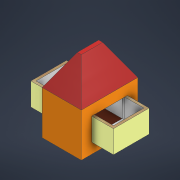
# Autodesk Inventor part: 110033226_ipt_55_內城堡屋頂
Saved by Autodesk Inventor 2022 (Build 260153000, 153)
## iProperties
Created: 2022-07-01
Part Number: 110033226_ipt_55_內城堡屋頂
Material: 一般
Document SubType Name: Modeling
Designer: User
Density: 1 g/cm^3
Appearance: 預設
Author: User
Autodesk Inventor part; units mm, degrees
ref_plane "YZ Plane" through (0, 0, 0) normal (1, 0, 0) x (0, 1, 0)
ref_plane "XZ Plane" through (0, 0, 0) normal (0, 1, 0) x (-1, 0, 0)
sketch "草圖1" plane through (0, 0, 0) normal (0, 1, 0) x (-1, 0, 0)
  line L0 (0, 0) -> (45, 0)
  line L1 (45, 0) -> (45, -65)
  line L2 (45, -65) -> (0, -65)
  line L3 (0, -65) -> (0, 0)
  dimension "d0" = 45
  dimension "d1" = 65
  constraints: 8 end point, 2 parallel, 1 horizontal, 1 perpendicular
  measures "d0" distance of L1.end L2.end
  measures "d1" distance of L0.end L1.end
extrude "擠出1" add sketch "草圖1" along normal blind 50
shell "薄殼1" thickness 3 removed faces 1 at (-15, 50, -21.666667)
sketch "草圖2" plane through (0, 0, 0) normal (1, 0, 0) x (0, 0, -1)
  line L0 (65, 50) -> (65, 0) projected
  line L1 (65, 0) -> (0, 0) projected
  line L2 (0, 0) -> (0, 50) projected
  line L3 (0, 50) -> (65, 50) projected
  line L4 (53, 38) -> (53, 12)
  line L5 (53, 12) -> (12, 12)
  line L6 (12, 12) -> (12, 38)
  line L7 (12, 38) -> (53, 38)
  dimension "d5" = 12
  constraints: 8 end point, 3 other
  measures "d5" distance between parallel lines of L3 L7
extrude "擠出2" add sketch "草圖2" along normal blind 25 separate body contours L4 L5 L6 L7
shell "薄殼2" thickness 3 removed faces 1 at (8.333333, 38, -39.333333) bodies 2
ref_plane "工作平面1" through (-22.5, 0, 0) normal (1, 0, 0) x (0, 0, -1)
sketch "草圖3" plane through (3, 15, -15) normal (1, 0, 0) x (0, 0, -1)
  line L0 (35, 0) -> (35, 23) projected
  line L1 (0, 23) -> (35, 23) projected
  line L2 (-3, 23) -> (0, 23) projected
  line L3 (-3, -3) -> (-3, 23) projected
  line L4 (38, -3) -> (-3, -3) projected
  line L5 (38, 23) -> (38, -3) projected
  line L6 (35, 23) -> (38, 23) projected
  line L7 (0, 0) -> (35, 0) projected
  line L8 (0, 23) -> (0, 0) projected
  point P0 (-15, -15)
extrude "擠出3" cut sketch "草圖3" against normal blind 25 contours L7 L8 L1 L0 bodies 2
sketch "草圖4" plane through (0, 0, 0) normal (1, 0, 0) x (0, 0, -1)
  line L0 (65, 50) -> (65, 0) projected
  line L1 (65, 0) -> (0, 0) projected
  line L2 (0, 0) -> (0, 50) projected
  line L3 (0, 50) -> (65, 50) projected
  line L4 (50, 38) -> (53, 38) projected
  line L5 (53, 38) -> (53, 12) projected
  line L6 (53, 12) -> (12, 12) projected
  line L7 (12, 12) -> (12, 38) projected
  line L8 (12, 38) -> (15, 38) projected
  line L9 (15, 38) -> (15, 15) projected
  line L10 (15, 15) -> (50, 15) projected
  line L11 (50, 15) -> (50, 38) projected
  line L12 (15, 38) -> (50, 38)
  line L13 (50, 38) -> (50, 15)
  line L14 (50, 15) -> (15, 15)
  line L15 (15, 15) -> (15, 38)
  constraints: 8 end point, 2 parallel, 1 horizontal, 1 perpendicular
extrude "擠出4" cut sketch "草圖4" against normal blind 10 contours L11 L10 L9 L12 bodies 1
mirror "鏡射1" about plane through (-22.5, 0, 0) normal (1, 0, 0) of "擠出4", "擠出2", "擠出3" bodies 1
shell "薄殼3" thickness 3 removed faces 1 at (-62.666667, 38, -26.666667) bodies 1
sketch "草圖5" plane through (-51, 15, -15) normal (-1, 0, 0) x (0, 0, 1)
  line L0 (0, 0) -> (0, 23) projected
  line L1 (-35, 23) -> (0, 23) projected
  line L2 (-38, 23) -> (-35, 23) projected
  line L3 (-38, -3) -> (-38, 23) projected
  line L4 (3, -3) -> (-38, -3) projected
  line L5 (3, 23) -> (3, -3) projected
  line L6 (0, 23) -> (3, 23) projected
  line L7 (-35, 0) -> (0, 0) projected
  line L8 (-35, 23) -> (-35, 0) projected
  point P0 (15, -15)
extrude "擠出5" cut sketch "草圖5" against normal blind 10 contours L7 L8 L1 L0 bodies 1
sketch "草圖6" plane through (0, 50, 0) normal (0, 1, 0) x (1, 0, 0)
  line L0 (-3, 3) -> (-3, 62) projected
  line L1 (-3, 62) -> (-42, 62) projected
  line L2 (-42, 62) -> (-42, 3) projected
  line L3 (-42, 3) -> (-3, 3) projected
  line L4 (0, 65) -> (0, 0) projected
  line L5 (0, 0) -> (-45, 0) projected
  line L6 (-45, 0) -> (-45, 65) projected
  line L7 (-45, 65) -> (0, 65) projected
sketch "草圖6 outline for 擠出6" plane through (0, 50, 0) normal (0, 1, 0) x (1, 0, 0)
  line L0 (0, 65) -> (-45, 65)
  line L1 (0, 0) -> (0, 65)
  line L2 (-45, 0) -> (0, 0)
  line L3 (-45, 65) -> (-45, 0)
extrude "擠出6" add sketch "草圖6 outline for 擠出6" along normal blind 35 draft -30 bodies 1
